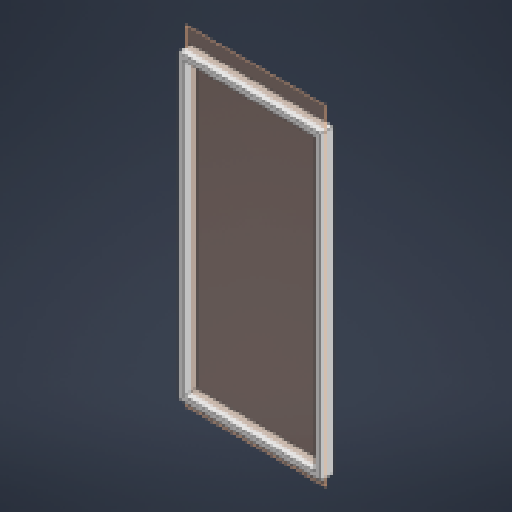
# Autodesk Inventor part: DoorFrame
Saved by Autodesk Inventor 2025.1 (Build 291241020, 241B)
## iProperties
Created: 2026-03-06
Part Number: DoorFrame
Material: Generic
Document SubType Name: Modeling
Designer: brand
Density: 1 g/cm^3
Appearance: Default
Author: brand
Autodesk Inventor part; units mm, degrees
ref_plane "YZ Plane" through (0, 0, 0) normal (1, 0, 0) x (0, 1, 0)
ref_plane "XZ Plane" through (0, 0, 0) normal (0, 1, 0) x (-1, 0, 0)
ref_plane "XY Plane" through (0, 0, 0) normal (0, 0, 1) x (1, 0, 0)
ref_plane "Work Plane1" through (0, 0, 0) normal (0, 0, 1) x (1, 0, 0)
sketch "Sketch1" plane through (0, 0, 0) normal (0, 0, 1) x (1, 0, 0)
  line L0 (-155.575, -1057.275) -> (454.025, -1057.275) projected
  line L1 (454.025, -1057.275) -> (454.025, 974.725) projected
  circle A0 centre (384.175, -28.575) radius 31.4325 projected
  line L2 (454.025, 1057.275) -> (-454.025, 1057.275)
  line L3 (-454.025, 1057.275) -> (-454.025, -1057.275)
  line L4 (-454.025, -1057.275) -> (454.025, -1057.275)
  line L5 (454.025, -1057.275) -> (454.025, 1057.275)
  line L6 (-200.025, 1019.175) -> (498.475, 1019.175)
  line L7 (498.475, 1019.175) -> (498.475, -1063.625)
  line L8 (498.475, -1063.625) -> (-200.025, -1063.625)
  line L9 (-200.025, -1063.625) -> (-200.025, 1019.175)
  line L10 (-463.55, 107.95) -> (-463.55, 825.5)
  line L11 (-463.55, 825.5) -> (-458.978, 825.5)
  line L12 (-458.978, 825.5) -> (-458.978, 930.275)
  line L13 (-458.978, 930.275) -> (-161.925, 930.275)
  line L14 (-161.925, 930.275) -> (-161.925, 981.075)
  line L15 (-161.925, 981.075) -> (460.375, 981.075)
  line L16 (460.375, 981.075) -> (460.375, -1063.625)
  line L17 (460.375, -1063.625) -> (-463.55, -1063.625)
  line L18 (-463.55, -1063.625) -> (-463.55, -812.8)
  line L19 (-463.55, -812.8) -> (-458.978, -812.8)
  line L20 (-458.978, -812.8) -> (-458.978, -711.2)
  line L21 (-458.978, -711.2) -> (-463.55, -711.2)
  line L22 (-463.55, -711.2) -> (-463.55, 6.35)
  line L23 (-463.55, 6.35) -> (-458.978, 6.35)
  line L24 (-458.978, 6.35) -> (-458.978, 107.95)
  line L25 (-458.978, 107.95) -> (-463.55, 107.95)
  line L26 (-161.925, 981.075) -> (460.375, 981.075)
  line L27 (460.375, 981.075) -> (460.375, -1063.625)
  line L28 (460.375, -1063.625) -> (-161.925, -1063.625)
  line L29 (-161.925, -1063.625) -> (-161.925, 981.075)
  line L30 (-200.025, -1063.625) -> (498.475, -1063.625)
  line L31 (498.475, -1063.625) -> (498.475, -1101.725)
  line L32 (498.475, -1101.725) -> (-200.025, -1101.725)
  line L33 (-200.025, -1101.725) -> (-200.025, -1063.625)
  line L34 (454.025, 974.725) -> (-155.575, 974.725) projected
  line L35 (-155.575, 974.725) -> (-155.575, -1057.275) projected
  point P0 (0, 0)
  point P1 (-463.55, -1063.625)
  point P2 (460.375, -1063.625)
  point P3 (-463.55, -815.975)
  point P4 (-463.55, -714.375)
  point P5 (-463.55, 3.175)
  point P6 (-463.55, 104.775)
  point P7 (-463.55, 822.325)
  point P8 (-200.025, 930.275)
  dimension "d1" = 38.1
  dimension "d2" = 38.1
  dimension "d3" = 38.1
  dimension "d10" = 38.1
  dimension "d11" = 6.35
  dimension "d12" = 6.35
  dimension "d13" = 6.35
  dimension "d14" = 6.35
  constraints: 64 end point, 8 parallel, 4 horizontal, 4 perpendicular, 1 other
  measures "d1" distance between parallel lines of L9 L14
  measures "d2" distance between parallel lines of L7 L16
  measures "d3" distance between parallel lines of L6 L15
  measures "d10" distance between parallel lines of L8 L32
  measures "d11" distance between parallel lines of L4 L8
  measures "d12" distance between parallel lines of L35 L29
  measures "d13" distance between parallel lines of L15 L34
  measures "d14" distance between parallel lines of L16 L1
extrude "Extrusion1" add sketch "Sketch1" along normal blind 95.25 and the other way blind 44.45 contours L29 L8 L9 L4 | L4 L9 L13 L29 | L8 L31 L32 L33 | L13 L9 L6 L5 L15 L14 | L5 L6 L7 L8 L16 L15
body "Solid1"
